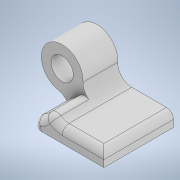
# Autodesk Inventor part: zawias
Saved by Autodesk Inventor 2021 (Build 250183000, 183)
## iProperties
Created: 2022-02-09
Part Number: zawias
Material: Generic
Document SubType Name: Modeling
Designer: Łukasz
Density: 1 g/cm^3
Appearance: Default
Author: Łukasz
Autodesk Inventor part; units mm, degrees
ref_plane "YZ Plane" through (0, 0, 0) normal (1, 0, 0) x (0, 1, 0)
ref_plane "XZ Plane" through (0, 0, 0) normal (0, 1, 0) x (-1, 0, 0)
ref_plane "XY Plane" through (0, 0, 0) normal (0, 0, 1) x (1, 0, 0)
sketch "Sketch1" plane through (0, 0, 0) normal (0, 0, 1) x (1, 0, 0)
  circle A0 centre (0, 0) radius 1.6
  circle A1 centre (0, 0) radius 3
  line L0 (1, -2.8284) -> (1, -4.3284)
  line L1 (1, -2.8284) -> (2.5, -2.8284) construction
  line L2 (1, -4.3284) -> (11, -4.3284)
  line L3 (11, -4.3284) -> (11, -2.3284)
  line L4 (11, -2.3284) -> (1.8917, -2.3284)
  dimension "d0" = 3.2
  dimension "d1" = 6
  dimension "d2" = 1.5
  dimension "d3" = 90
  dimension "d4" = 10
  dimension "d5" = 2
  constraints: 10 end point, 4 perpendicular, 2 centre point, 2 coincident, 2 point on circle, 1 horizontal, 1 vertical
  measures "d0" diameter of A0
  measures "d1" diameter of A1
  measures "d2" distance of L0.start L0.end
  measures "d3" angle of L0 L1
  measures "d4" distance of L0.end L2.end
  measures "d5" distance of L2.end L3.end
extrude "Extrusion1" add sketch "Sketch1" along normal blind 5
fillet "Fillet1" radius 2 2 edges at (1.8917, -2.3284, 2.5) (1, -2.8284, 2.5)
sketch "Sketch2" plane through (0, 0, 5) normal (0, 0, 1) x (1, 0, 0)
  circle A0 centre (0, 0) radius 1.6 projected
  circle A1 centre (0, 0) radius 3.25
  line L0 (11, -2.3284) -> (4.9892, -2.3284) projected
  arc A2 (2.9935, -0.1971) -> (4.9892, -2.3284) centre (4.9892, -0.3284) ccw projected
  arc A3 (2.9935, -0.1971) -> (-0.547, -2.9497) centre (0, 0) ccw projected
  arc A4 (1, -4.3284) -> (-0.547, -2.9497) centre (-0.9117, -4.9162) ccw projected
  line L1 (1, -4.3284) -> (11, -4.3284) projected
  line L2 (11, -4.3284) -> (11, -2.3284) projected
  circle A5 centre (0, 0) radius 1.6 projected
  point P0 (3.0985, -0.9806)
  point P1 (0.1865, -3.2446)
  dimension "d9" = 6.5
  constraints: 1 centre point, 1 coincident
  measures "d9" diameter of A1
extrude "Extrusion2" add sketch "Sketch2" along normal blind 5 contours A1 A2 L0 L2 L1 A4
fillet "Fillet2" radius 1 2 edges at (3.0985, -0.9806, 7.5) (0.1865, -3.2446, 7.5)
fillet "Fillet3" radius 1 7 edges at (7.9946, -2.3284, 10) (4.3736, -2.2313, 10) (3.1131, -1.767, 10) (1.9948, -2.5658, 10) (0.945, -3.4526, 10) (0.9755, -4.2539, 10) (11, -2.3284, 5)
body "Solid1"
